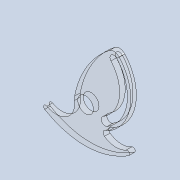
# Autodesk Inventor part: スライダヘッケン
Saved by Autodesk Inventor 2020 (Build 240168000, 168)
## iProperties
Created: 2020-10-30
Part Number: スライダヘッケン
Material: ポリカーボネート、クリア
Document SubType Name: Modeling
Designer: AA19065
Density: 1.2 g/cm^3
Appearance: ポリカーボネート - クリア
Author: AA19065
Autodesk Inventor part; units mm, degrees
ref_plane "YZ Plane" through (0, 0, 0) normal (1, 0, 0) x (0, 1, 0)
ref_plane "XZ Plane" through (0, 0, 0) normal (0, 1, 0) x (-1, 0, 0)
ref_plane "XY Plane" through (0, 0, 0) normal (0, 0, 1) x (1, 0, 0)
sketch "スケッチ1" plane through (0, 0, 0) normal (0, 0, 1) x (1, 0, 0)
  spline S0 degree 4 poles (38.5164, -45.3071) (32.8481, -48.7398) (24.8697, -52.6693) (14.1951, -56.043) (0.8314, -57.2802) (-12.4856, -56.5839) (-23.1422, -53.6497) (-31.0469, -50.0387) (-36.604, -46.8264) knots 0 0 0 0 0 0.316504 0.440375 0.563623 0.687019 1 1 1 1 1
  arc A0 (-34.6019, -43.3635) -> (-36.604, -46.8264) centre (-35.6029, -45.0949) ccw
  arc A1 (38.5164, -45.3071) -> (36.4435, -41.8861) centre (37.48, -43.5966) ccw
  arc A2 (-34.6019, -43.3635) -> (-9.8865, -26.5022) centre (-26.2949, -28.9953) ccw
  arc A3 (9.9747, -25.7104) -> (36.4435, -41.8861) centre (27.3937, -26.9509) ccw
  circle A4 centre (0, -25) radius 10
  circle A5 centre (0, -25) radius 7.025
  line L0 (0, 0) -> (0, -25) construction
  line L1 (0, -25) -> (8.9317, -40.6277) construction
  line L2 (8.9317, -40.6277) -> (31.5659, -12.6331) construction
  line L3 (31.5659, -12.6331) -> (0, 0) construction
  circle A6 centre (25.3122, 22.7) radius 3.5
  circle A7 centre (17.5174, -29.14) radius 3.5
  arc A8 (15.7142, -26.1403) -> (22.7066, 20.3632) centre (0, 0) ccw
  arc A9 (19.3207, -32.1397) -> (27.9179, 25.0368) centre (0, 0) ccw
  circle A10 centre (31.5659, -12.6331) radius 3 construction
  arc A11 (14.1685, -23.5691) -> (20.4731, 18.3603) centre (0, 0) ccw
  arc A12 (20.8664, -34.7109) -> (30.1514, 27.0397) centre (0, 0) ccw
  circle A13 centre (25.3122, 22.7) radius 6.5
  circle A14 centre (17.5174, -29.14) radius 6.5
  arc A15 (21.3095, 27.8213) -> (-9.8204, -23.1133) centre (73.6531, -39.1499) ccw
  arc A16 (18.3707, -35.5837) -> (16.9747, -40.9653) centre (18.7646, -38.5578) ccw
  point P0 (29.1445, -50.2982)
  point P1 (19.8001, -53.8831)
  point P2 (10.3498, -56.1165)
  point P3 (0.8079, -56.9906)
  point P4 (-8.734, -56.4935)
  point P5 (-18.1675, -54.6313)
  point P6 (-27.4303, -51.4198)
  point P7 (30.1514, 27.0397)
  dimension "d0" = 18
  dimension "d1" = 36
  dimension "d2" = 34
  dimension "d3" = 7
  dimension "d4" = 6
  dimension "d5" = 3
  dimension "d6" = 3
  dimension "d7" = 3
  dimension "d8" = 3
  dimension "d9" = 85
  dimension "d10" = 3
  constraints: 26 point on circle, 15 centre point, 8 end point, 4 tangent, 3 coincident, 2 vertical, 1 equal radius, 33 other
  measures "d0" distance of L0.end L1.end
  measures "d1" distance of L1.end L2.end
  measures "d2" distance of L2.end L0.start
  measures "d3" diameter of A6
  measures "d4" diameter of A10
  measures "d5" radial gap between concentric circles of A8 A11
  measures "d6" radial gap between concentric circles of A9 A12
  measures "d9" radius of A15
  measures "d10" radius of A16
extrude "押し出し1" add sketch "スケッチ1" along normal blind 5 contours S0 A0 A2 A4 A3 A1 | A3 A4 A15 A13 A11 A14 A16 | A4 | A14 A8 A7 A9 | A11 A13 A8 A14 | A14 A9 A13 A12 | A13 A9 A6 A8 picked at (20.7316, -32.3858) picked at (29.3785, 24.7855)
equation "\"d0\" = d11"
equation "\"d1\" = d12"
equation "\"d2\" = d13"
equation "\"d11\" = 18"
equation "\"d12\" = 36"
equation "\"d13\" = 34"
